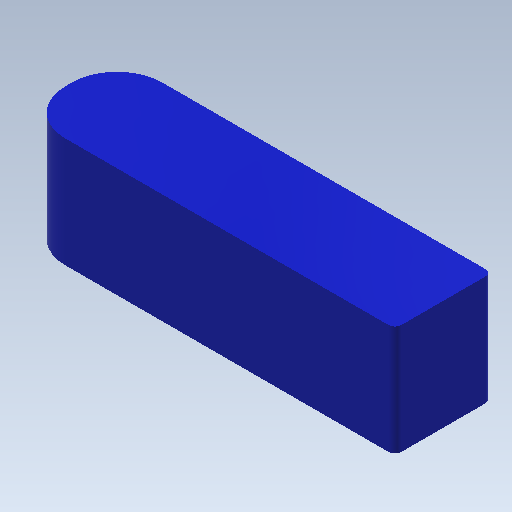
# Autodesk Inventor part: HP-G570-2600S3
Saved by Autodesk Inventor 2020.4 (Build 244396000, 396)
## iProperties
Created: 2016-05-03
Part Number: HP-G570-2600S3
Material: 一般
Document SubType Name: Modeling
Designer: Masato Kubotera
Mass: 220 g
Surface Area: 165.276 cm^2
Volume: 118.796 cm^3
Density: 1.85192 g/cm^3
Appearance: 青 - 壁塗料 - 光沢
Description: 既製品
Author: Masato Kubotera
Title: HP-G570-2600S3
Autodesk Inventor part; units mm, degrees
ref_plane "YZ Plane" through (0, 0, 0) normal (1, 0, 0) x (0, 1, 0)
ref_plane "XZ Plane" through (0, 0, 0) normal (0, 1, 0) x (-1, 0, 0)
ref_plane "XY Plane" through (0, 0, 0) normal (0, 0, 1) x (1, 0, 0)
sketch "スケッチ1" plane through (0, 0, 0) normal (0, 0, 1) x (1, 0, 0)
  line L0 (-58, -17) -> (58, -17)
  line L1 (58, -17) -> (58, 17)
  line L2 (58, 17) -> (-58, 17)
  line L3 (-58, 17) -> (-58, -17)
  line L4 (-58, -17) -> (58, 17) construction
  line L5 (58, -17) -> (-58, 17) construction
  point P0 (0, 0)
  dimension "d0" = 116
  dimension "d1" = 34
  constraints: 12 end point, 2 midpoint, 2 parallel, 1 horizontal, 1 perpendicular
  measures "d0" distance of L1.end L2.end
  measures "d1" distance of L0.end L1.end
extrude "押し出し1" add sketch "スケッチ1" along normal blind 15
mirror "ミラー1" about plane through (0, 0, 0) normal (0, 0, -1) of "押し出し1"
fillet "フィレット1" radius 14 2 edges at (-58, 0, 15) (-58, 0, -15)
fillet "フィレット2" radius 2 2 edges at (58, 0, 15) (58, 0, -15)
